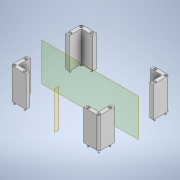
# Autodesk Inventor part: enclosure corner standoffs
Saved by Autodesk Inventor 2022 (Build 260153000, 153)
## iProperties
Created: 2021-11-30
Part Number: enclosure corner standoffs
Material: Generic
Document SubType Name: Modeling
Designer: a-dubs
Density: 1 g/cm^3
Appearance: Default
Author: a-dubs
Autodesk Inventor part; units mm, degrees
ref_plane "YZ Plane" through (0, 0, 0) normal (1, 0, 0) x (0, 1, 0)
ref_plane "XZ Plane" through (0, 0, 0) normal (0, 1, 0) x (-1, 0, 0)
ref_plane "XY Plane" through (0, 0, 0) normal (0, 0, 1) x (1, 0, 0)
sketch "Sketch1" plane through (0, 0, 0) normal (0, 1, 0) x (-1, 0, 0)
  line L0 (0, 0) -> (61, 0)
  circle A0 centre (0, 0) radius 33.6
  circle A1 centre (61, 0) radius 8.05
  line L1 (69.05, 0) -> (69.05, 7.5)
  line L2 (69.05, 7.5) -> (69.05, -7.5)
  line L3 (69.05, -7.5) -> (63.9245, -7.5)
  line L4 (69.05, 7.5) -> (63.9245, 7.5)
  line L5 (69.05, 7.5) -> (72.05, 7.5)
  line L6 (72.05, 7.5) -> (72.05, -7.5)
  line L7 (72.05, -7.5) -> (69.05, -7.5)
  line L8 (52.95, 0) -> (47.95, 0)
  line L9 (61, 8.05) -> (61, 13.05)
  line L10 (72.05, 0) -> (77.05, 0)
  line L11 (61, -8.05) -> (61, -13.05)
  line L12 (47.95, 13.05) -> (77.05, 13.05)
  line L13 (77.05, 13.05) -> (77.05, -13.05)
  line L14 (77.05, -13.05) -> (47.95, -13.05)
  line L15 (47.95, -13.05) -> (47.95, 13.05)
  line L16 (72.05, 7.5) -> (72.05, 10.5)
  line L17 (72.05, 10.5) -> (63.9245, 10.5)
  line L18 (63.9245, 10.5) -> (63.9245, 7.5)
  line L19 (72.05, -7.5) -> (72.05, -10.5)
  line L20 (72.05, -10.5) -> (63.9245, -10.5)
  line L21 (63.9245, -10.5) -> (63.9245, -7.5)
  line L22 (61, 0) -> (61, 60)
  line L23 (0, 0) -> (-42.65, 0)
  line L24 (-42.65, 0) -> (-47.65, 0)
  line L25 (0, 0) -> (0, -33.6)
  line L26 (0, 0) -> (42.65, 0)
  line L27 (42.65, 0) -> (42.65, 60)
  line L28 (42.65, 0) -> (42.65, -33.6)
  circle A2 centre (61, 0) radius 25
  line L29 (42.65, 25) -> (42.65, 31.2)
  line L30 (42.65, 31.2) -> (48.85, 31.2)
  line L31 (42.65, -25) -> (42.65, -31.2)
  line L32 (42.65, -31.2) -> (48.85, -31.2)
  circle A3 centre (48.85, 31.2) radius 3.1
  circle A4 centre (48.85, 31.2) radius 1.6
  circle A5 centre (48.85, 31.2) radius 1.45
  circle A6 centre (48.85, -31.2) radius 3.1
  circle A7 centre (48.85, -31.2) radius 1.6
  circle A8 centre (48.85, -31.2) radius 1.45
  circle A9 centre (73.15, 31.2) radius 3.1
  circle A10 centre (73.15, 31.2) radius 1.6
  circle A11 centre (73.15, 31.2) radius 1.45
  circle A12 centre (73.15, -31.2) radius 3.1
  circle A13 centre (73.15, -31.2) radius 1.45
  circle A14 centre (73.15, -31.2) radius 1.6
  line L33 (73.15, 31.2) -> (79.35, 31.2)
  line L34 (73.15, -31.2) -> (79.35, -31.2)
  line L35 (36, 0) -> (31, 0)
  line L36 (31, 0) -> (31, -31.2)
  line L37 (31, -31.2) -> (31, -37.4)
  line L38 (31, -37.4) -> (79.35, -37.4)
  line L39 (79.35, -37.4) -> (79.35, 31.2)
  line L40 (79.35, 31.2) -> (79.35, 37.4)
  line L41 (79.35, 37.4) -> (31, 37.4)
  line L42 (31, 37.4) -> (31, 0)
  line L43 (42.65, -33.6) -> (42.65, -37.4)
  circle A15 centre (61, 0) radius 5.25
  line L44 (86, 0) -> (91, 0)
  line L45 (91, 0) -> (97.4, 0)
  line L46 (-47.65, 0) -> (-47.65, 60)
  line L47 (-47.65, 60) -> (42.65, 60)
  line L48 (91, 0) -> (91, 60)
  line L49 (91, 60) -> (42.65, 60)
  line L50 (0, -33.6) -> (0, -43.6)
  line L51 (0, -43.6) -> (0, -48.6)
  line L52 (0, -48.6) -> (0, -55)
  line L53 (0, -55) -> (-54.05, -55)
  line L54 (0, -48.6) -> (-47.65, -48.6)
  line L55 (-47.65, -48.6) -> (-47.65, 0)
  line L56 (0, -55) -> (97.4, -55)
  line L57 (97.4, -55) -> (97.4, 0)
  line L58 (91, 0) -> (91, -48.6)
  line L59 (91, -48.6) -> (0, -48.6)
  line L60 (0, -48.6) -> (10, -48.6)
  line L61 (0, -48.6) -> (-10, -48.6)
  line L62 (10, -48.6) -> (10, -55)
  line L63 (-10, -48.6) -> (-10, -55)
  line L64 (10, -48.6) -> (10, -43.6)
  line L65 (10, -43.6) -> (-10, -43.6)
  line L66 (-10, -43.6) -> (-10, -49.0563)
  line L67 (63.9245, 10.5) -> (64.9245, 10.5)
  line L68 (64.9245, 10.5) -> (64.9245, 7.5)
  line L69 (63.9245, -10.5) -> (64.9245, -10.5)
  line L70 (64.9245, -10.5) -> (64.9245, -7.5)
  line L71 (-47.65, 0) -> (-54.05, 0)
  line L72 (42.65, 60) -> (42.65, 66.4)
  line L73 (-54.05, -55) -> (-54.05, 0)
  line L74 (-54.05, 66.4) -> (-54.05, 0)
  line L75 (42.65, 66.4) -> (-54.05, 66.4)
  line L76 (97.4, 0) -> (97.4, 66.4)
  line L77 (97.4, 66.4) -> (42.65, 66.4)
  line L78 (-47.65, 60) -> (-50.85, 60)
  line L79 (-50.85, 60) -> (-50.85, 63.2)
  circle A16 centre (-50.85, 63.2) radius 1.6
  line L80 (91, 60) -> (94.2, 60)
  line L81 (94.2, 60) -> (-50.85, 60)
  circle A17 centre (-32.7188, 63.2) radius 1.6
  circle A18 centre (-14.5875, 63.2) radius 1.6
  circle A19 centre (3.5438, 63.2) radius 1.6
  circle A20 centre (21.675, 63.2) radius 1.6
  circle A21 centre (39.8063, 63.2) radius 1.6
  circle A22 centre (57.9375, 63.2) radius 1.6
  circle A23 centre (76.0688, 63.2) radius 1.6
  circle A24 centre (94.2, 63.2) radius 1.6
  line L82 (-47.65, 60) -> (-47.65, 63.2)
  line L83 (-47.65, 63.2) -> (-47.65, -51.8)
  circle A25 centre (-50.85, 44.0333) radius 1.6
  circle A26 centre (-50.85, 24.8667) radius 1.6
  circle A27 centre (-50.85, 5.7) radius 1.6
  circle A28 centre (-50.85, -13.4667) radius 1.6
  circle A29 centre (-50.85, -32.6333) radius 1.6
  circle A30 centre (-50.85, -51.8) radius 1.6
  line L84 (-47.65, 60) -> (21.675, 60)
  line L85 (21.675, 60) -> (21.675, 55.1722)
  line L86 (-47.65, 5.7) -> (-45.15, 5.7)
  circle A31 centre (-50.85, -51.8) radius 1.6
  circle A32 centre (-32.7188, -51.8) radius 1.6
  circle A33 centre (-14.5875, -51.8) radius 1.6
  circle A34 centre (3.5438, -51.8) radius 1.6
  circle A35 centre (21.675, -51.8) radius 1.6
  circle A36 centre (39.8063, -51.8) radius 1.6
  circle A37 centre (57.9375, -51.8) radius 1.6
  circle A38 centre (76.0688, -51.8) radius 1.6
  circle A39 centre (94.2, -51.8) radius 1.6
  circle A40 centre (94.2, 44.0333) radius 1.6
  circle A41 centre (94.2, 24.8667) radius 1.6
  circle A42 centre (94.2, 5.7) radius 1.6
  circle A43 centre (94.2, -13.4667) radius 1.6
  circle A44 centre (94.2, -32.6333) radius 1.6
  line L87 (61, 60) -> (61, 56.8)
  line L88 (61, 56.8) -> (61, 39)
  line L89 (61, 56.8) -> (48.1, 56.8)
  line L90 (61, 56.8) -> (73.9, 56.8)
  line L91 (73.9, 56.8) -> (73.9, 39)
  line L92 (73.9, 39) -> (61, 39)
  line L93 (48.1, 56.8) -> (48.1, 39)
  line L94 (48.1, 39) -> (61, 39)
  line L95 (0, 60) -> (0, 56.8)
  line L96 (0, 56.8) -> (-16.55, 56.8)
  line L97 (-16.55, 56.8) -> (16.55, 56.8)
  line L98 (16.55, 56.8) -> (16.55, 38.6)
  line L99 (16.55, 38.6) -> (-16.55, 38.6)
  line L100 (-16.55, 38.6) -> (-16.55, 56.8)
  circle A45 centre (-50.85, 63.2) radius 1.4
  circle A46 centre (-32.7188, 63.2) radius 1.4
  circle A47 centre (-14.5875, 63.2) radius 1.4
  circle A48 centre (3.5438, 63.2) radius 1.4
  circle A49 centre (21.675, 63.2) radius 1.4
  circle A50 centre (39.8063, 63.2) radius 1.4
  circle A51 centre (57.9375, 63.2) radius 1.4
  circle A52 centre (76.0688, 63.2) radius 1.4
  circle A53 centre (94.2, 63.2) radius 1.4
  circle A54 centre (-50.85, -51.8) radius 1.4
  circle A55 centre (-32.7188, -51.8) radius 1.4
  circle A56 centre (-14.5875, -51.8) radius 1.4
  circle A57 centre (3.5438, -51.8) radius 1.4
  circle A58 centre (21.675, -51.8) radius 1.4
  circle A59 centre (39.8063, -51.8) radius 1.4
  circle A60 centre (57.9375, -51.8) radius 1.4
  circle A61 centre (76.0688, -51.8) radius 1.4
  circle A62 centre (94.2, -51.8) radius 1.4
  circle A63 centre (-50.85, 44.0333) radius 1.4
  circle A64 centre (-50.85, 24.8667) radius 1.4
  circle A65 centre (-50.85, 5.7) radius 1.4
  circle A66 centre (-50.85, -13.4667) radius 1.4
  circle A67 centre (-50.85, -32.6333) radius 1.4
  circle A68 centre (-50.85, -51.8) radius 1.4
  circle A69 centre (94.2, 63.2) radius 1.4
  circle A70 centre (94.2, 44.0333) radius 1.4
  circle A71 centre (94.2, 24.8667) radius 1.4
  circle A72 centre (94.2, 5.7) radius 1.4
  circle A73 centre (94.2, -13.4667) radius 1.4
  circle A74 centre (94.2, -32.6333) radius 1.4
  circle A75 centre (94.2, -51.8) radius 1.4
  line L101 (-50.85, 44.0333) -> (-50.85, 24.8667)
  line L102 (-50.85, 24.8667) -> (-50.85, 34.45)
  circle A76 centre (-50.85, 63.2) radius 3.2
  circle A77 centre (-50.85, -51.8) radius 3.2
  circle A78 centre (94.2, -51.8) radius 3.2
  circle A79 centre (94.2, 63.2) radius 3.2
  line L103 (-50.85, 34.45) -> (-54.05, 34.45)
  line L104 (-47.65, 34.45) -> (-50.85, 34.45)
  line L105 (-31.3187, 63.2) -> (-16.1875, 63.2)
  line L106 (-31.1187, 63.2) -> (-27.9188, 63.2)
  line L107 (-27.9188, 63.2) -> (-27.9188, 60)
  line L108 (-27.9188, 63.2) -> (-27.9188, 66.4)
  line L109 (-50.85, 42.4333) -> (-50.85, 39.2333)
  line L110 (-50.85, 39.2333) -> (-47.65, 39.2333)
  line L111 (-54.05, 39.2333) -> (-50.85, 39.2333)
  point P0 (42.65, 37.4)
  point P1 (31, -12.9599)
  point P2 (31, 12.9599)
  point P3 (-23.7531, 63.2)
  point P4 (-23.7031, 66.4)
  point P5 (-50.85, 66.4)
  point P6 (-54.05, 63.2)
  dimension "d1" = 67.2
  dimension "d0" = 61
  dimension "d2" = 16.1
  dimension "d3" = 7.5
  dimension "d4" = 15
  dimension "d5" = 3
  dimension "d6" = 5
  dimension "d7" = 5
  dimension "d8" = 5
  dimension "d9" = 5
  dimension "d10" = 3
  dimension "d11" = 60
  dimension "d13" = 42.65
  dimension "d14" = 5
  dimension "d16" = 50
  dimension "d17" = 6.2
  dimension "d18" = 6.2
  dimension "d19" = 6.2
  dimension "d20" = 6.2
  dimension "d21" = 6.2
  dimension "d22" = 3.2
  dimension "d23" = 2.9
  dimension "d24" = 6.2
  dimension "d25" = 6.2
  dimension "d26" = 5
  dimension "d27" = 6.2
  dimension "d28" = 6.2
  dimension "d31" = 10.5
  dimension "d33" = 5
  dimension "d34" = 6.4
  dimension "d36" = 10
  dimension "d37" = 5
  dimension "d38" = 6.4
  dimension "d41" = 10
  dimension "d42" = 10
  dimension "d52" = 1
  dimension "d53" = 1
  dimension "d56" = 6.4
  dimension "d57" = 6.4
  dimension "d58" = 3.2
  dimension "d59" = 3.2
  dimension "d62" = 18.1313
  dimension "d67" = 115
  dimension "d70" = 19.1667
  dimension "d78" = 3.2
  dimension "d79" = 17.8
  dimension "d80" = 12.9
  dimension "d81" = 12.9
  dimension "d82" = 3.2
  dimension "d83" = 16.55
  dimension "d84" = 33.1
  dimension "d85" = 18.2
  dimension "d93" = 2.8
  dimension "d96" = 18.1313
  dimension "d99" = 115
  dimension "d104" = 19.1667
  dimension "d107" = 145.05
  dimension "d110" = 6.4
  dimension "d111" = 6.4
  dimension "d112" = 6.4
  dimension "d113" = 6.4
  dimension "d122" = 3.2
  dimension "d123" = 3.2
  constraints: 224 end point, 75 centre point, 47 point on line, 33 perpendicular, 26 symmetric about line, 21 vertical, 20 coincident, 20 horizontal, 8 point on circle, 7 parallel, 5 collinear, 5 midpoint, 3 horizontal alignment, 1 vertical alignment, 121 other
  measures "d0" distance of L0.start L0.end
  measures "d2" diameter of A1
  measures "d3" distance of L1.start L1.end
  measures "d4" distance of L1.end L2.end
  measures "d5" distance of L1.end L5.end
  measures "d6" distance of L8.start L8.end
  measures "d7" distance of L9.start L9.end
  measures "d8" distance of L10.start L10.end
  measures "d9" distance of L11.start L11.end
  measures "d10" distance of L5.end L16.end
  measures "d11" distance of L22.start L22.end
  measures "d13" distance of L23.start L23.end
  measures "d14" distance of L23.end L24.end
  measures "d16" diameter of A2
  measures "d17" distance of L29.start L29.end
  measures "d18" distance of L29.end L30.end
  measures "d19" distance of L31.start L31.end
  measures "d20" distance of L31.end L32.end
  measures "d21" diameter of A3
  measures "d22" diameter of A4
  measures "d23" diameter of A5
  measures "d24" distance of L33.start L33.end
  measures "d25" distance of L34.start L34.end
  measures "d26" distance of L35.start L35.end
  measures "d27" distance of L36.end L37.end
  measures "d28" distance of L33.end L40.end
  measures "d31" diameter of A15
  measures "d33" distance of L44.start L44.end
  measures "d34" distance of L44.end L45.end
  measures "d36" distance of L25.end L50.end
  measures "d37" distance of L50.end L51.end
  measures "d38" distance of L51.end L52.end
  measures "d41" distance of L51.end L60.end
  measures "d42" distance of L51.end L61.end
  measures "d52" distance of L17.end L67.end
  measures "d53" distance of L20.end L69.end
  measures "d56" distance of L24.end L71.end
  measures "d57" distance of L27.end L72.end
  measures "d58" distance of L46.end L78.end
  measures "d59" diameter of A16
  measures "d62" distance of A16.centre point (-32.719, 63.2)
  measures "d67" distance of L82.end L83.end
  measures "d70" distance of A16.centre point (-50.85, 44.033)
  measures "d78" distance of L22.end L87.end
  measures "d79" distance of L87.end L88.end
  measures "d80" distance of L87.end L89.end
  measures "d81" distance of L87.end L90.end
  measures "d82" distance of L95.start L95.end
  measures "d83" distance of L95.end L96.end
  measures "d84" distance of L96.end L97.end
  measures "d85" distance of L97.end L98.end
  measures "d93" diameter of A45
  measures "d96" distance of A45.centre point (-32.719, 63.2)
  measures "d99" distance of A45.centre A54.centre
  measures "d104" distance of A45.centre L101.start
  measures "d107" distance of A45.centre A69.centre
  measures "d110" diameter of A76
  measures "d111" diameter of A77
  measures "d112" diameter of A78
  measures "d113" diameter of A79
  measures "d122" distance of L106.start L106.end
  measures "d123" distance of L109.start L109.end
extrude "Extrusion12" add sketch "Sketch1" along normal blind 53 contours L110 L111 L74 A76 L78 L46 | L108 L107 L47 L82 A76 L75 | L78 A76 L82 | A76 | A16 | A17 | A25 | A45 | A46 | A63
extrude "Extrusion13" cut sketch "Sketch1" against normal blind 6.2 from surface at 53 contours A16 | A17 | A25 | A45 | A46 | A63
extrude "Extrusion14" add sketch "Sketch1" against normal blind 6 contours A45 | A46 | A63
fillet "Fillet8" radius 0.8 6 edges at (52.45, 53, 63.2) (52.25, 0, 63.2) (52.25, 0, 44.0333) (34.1187, 0, 63.2) (34.3187, 53, 63.2) (52.45, 53, 44.0333)
fillet "Fillet9" radius 1.4 3 edges at (52.25, -6, 63.2) (52.25, -6, 44.0333) (34.1187, -6, 63.2)
ref_plane "Work Plane1" through (-21.675, 0, 60) normal (1, 0, 0) x (0, 0, -1)
mirror "Mirror1" about plane through (-21.675, 0, 60) normal (1, 0, 0) of "Extrusion12", "Extrusion13", "Extrusion14", "Fillet8", "Fillet9"
ref_plane "Work Plane2" through (47.65, 0, 5.7) normal (0, 0, -1) x (-1, 0, 0)
mirror "Mirror2" about plane through (47.65, 0, 5.7) normal (0, 0, -1) of "Extrusion12", "Extrusion13", "Extrusion14", "Fillet8", "Fillet9", "Mirror1"
body "Solid4"
